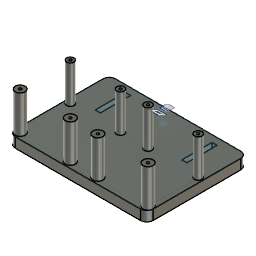
Halterung_BTS7960 (Autodesk Fusion 360 design; units mm, degrees)
part number: 2026-02-15-17-28-29-265
Autodesk Fusion 360 part; units mm, degrees
sketch "Skizze1" plane through (0, 0, 0) normal (0, 0, 1) x (1, 0, 0)
  line L0 (-35, 15) -> (50, 15)
  line L1 (50, 15) -> (50, -20)
  line L2 (50, -20) -> (-35, -20)
  line L3 (-35, -20) -> (-35, 15)
  dimension "d1" = 85
  dimension "d2" = 35
  constraint horizontal L0
  constraint vertical L1
  constraint horizontal L2
  constraint vertical L3
  measures "d1" distance of L0.start L0.end
  measures "d2" distance of L0 L2
extrude "Extrusion1" add sketch "Skizze1" along normal blind 8
sketch "Skizze2" plane through (0, 0, 8) normal (0, 0, 1) x (-1, 0, 0)
  line L0 (35, 20) -> (-50, 20)
  line L1 (-50, 20) -> (-50, -15)
  line L2 (-50, -15) -> (35, -15)
  line L3 (35, -15) -> (35, 20)
  line L4 (29, -9.5) -> (25, -9.5)
  line L5 (25, -9.5) -> (25, 14.5)
  line L6 (25, 14.5) -> (29, 14.5)
  line L7 (29, 14.5) -> (29, -9.5)
  line L8 (-40, -9.5) -> (-44, -9.5)
  line L9 (-44, -9.5) -> (-44, 14.5)
  line L10 (-44, 14.5) -> (-40, 14.5)
  line L11 (-40, 14.5) -> (-40, -9.5)
  dimension "d5" = 65
  dimension "d6" = 6
  dimension "d7" = 6
  dimension "d8" = 4
  dimension "d9" = 4
  dimension "d10" = 5.5
  dimension "d16" = 35
  dimension "d17" = 24
  dimension "d18" = 24
  dimension "d19" = 5.5
  dimension "d20" = 5.5
  constraint horizontal L4
  constraint vertical L5
  constraint horizontal L6
  constraint vertical L7
  constraint horizontal L8
  constraint vertical L9
  constraint horizontal L10
  constraint vertical L11
  measures "d5" distance of L5 L11
  measures "d6" distance of L3 L7
  measures "d7" distance of L1 L9
  measures "d8" distance of L9.end L10.end
  measures "d9" distance of L5.end L6.end
  measures "d10" distance of L0 L6
  measures "d16" distance of L0.start L2.end
  measures "d17" distance of L4 L6
  measures "d18" distance of L8.end L9.end
  measures "d19" distance of L0 L10
  measures "d20" distance of L2 L8
extrude "Extrusion2" cut sketch "Skizze2" against normal blind 8 contours L4 L5 L6 L7 | L8 L9 L10 L11
sketch "Skizze3" plane through (0, 0, 8) normal (0, 0, 1) x (-1, 0, 0)
  line L0 (25, -9.5) -> (25, 14.5)
  line L1 (25, 14.5) -> (29, 14.5)
  line L2 (29, 14.5) -> (29, -9.5)
  line L3 (29, -9.5) -> (25, -9.5)
  line L4 (-44, -9.5) -> (-44, 14.5)
  line L5 (-44, 14.5) -> (-40, 14.5)
  line L6 (-40, 14.5) -> (-40, -9.5)
  line L7 (-40, -9.5) -> (-44, -9.5)
  line L8 (35, 20) -> (-50, 20)
  line L9 (-50, 20) -> (-50, -15)
  line L10 (-50, -15) -> (35, -15)
  line L11 (35, -15) -> (35, 20)
  point P0 (-7.5, -3)
  dimension "d13" = 42.5
  dimension "d14" = 4
  dimension "d15" = 5.5
  dimension "d21" = 12
  measures "d13" distance of L11 P0
  measures "d14" distance of L0.start L2.end
  measures "d15" distance of L3 L10
  measures "d21" distance of L10 P0
hole "Bohrung1" at (7.5, 3, 8) direction (0, 0, -1) diameter 4 depth 25 tip angle 118
sketch "Skizze4" plane through (-35, 0, 0) normal (-1, 0, 0) x (0, -1, 0)
  line L0 (-15, 0) -> (20, 0)
  line L1 (20, 0) -> (20, 8)
  line L2 (20, 8) -> (-15, 8)
  line L3 (-15, 8) -> (-15, 0)
  line L4 (-15, 8) -> (20, 8)
  line L5 (20, 8) -> (20, 0)
  line L6 (20, 0) -> (-15, 0)
  line L7 (-15, 0) -> (-15, 8)
  constraint horizontal L4
  constraint vertical L5
  constraint horizontal L6
  constraint vertical L7
  constraint coincident L0.end L1.start
  constraint coincident L2.end L3.start
extrude "Extrusion3" add sketch "Skizze4" along normal blind 12.5
sketch "Skizze5" plane through (50, 0, 0) normal (1, 0, 0) x (0, 1, 0)
  line L0 (-20, 0) -> (15, 0)
  line L1 (15, 0) -> (15, 8)
  line L2 (15, 8) -> (-20, 8)
  line L3 (-20, 8) -> (-20, 0)
  line L4 (-20, 8) -> (15, 8)
  line L5 (15, 8) -> (15, 0)
  line L6 (15, 0) -> (-20, 0)
  line L7 (-20, 0) -> (-20, 8)
  constraint horizontal L4
  constraint vertical L5
  constraint horizontal L6
  constraint vertical L7
  constraint coincident L0.end L1.start
  constraint coincident L2.end L3.start
extrude "Extrusion4" add sketch "Skizze5" along normal blind 12.5
sketch "Skizze6" plane through (0, 0, 8) normal (0, 0, 1) x (-1, 0, 0)
  circle A0 centre (-7.5, -3) radius 2
  line L0 (25, -9.5) -> (25, 14.5)
  line L1 (25, 14.5) -> (29, 14.5)
  line L2 (29, 14.5) -> (29, -9.5)
  line L3 (29, -9.5) -> (25, -9.5)
  line L4 (-44, -9.5) -> (-44, 14.5)
  line L5 (-44, 14.5) -> (-40, 14.5)
  line L6 (-40, 14.5) -> (-40, -9.5)
  line L7 (-40, -9.5) -> (-44, -9.5)
sketch "Skizze7" plane through (0, -20, 0) normal (0, -1, 0) x (1, 0, 0)
  line L0 (-47.5, 0) -> (62.5, 0)
  line L1 (62.5, 0) -> (62.5, 8)
  line L2 (62.5, 8) -> (-47.5, 8)
  line L3 (-47.5, 8) -> (-47.5, 0)
  line L4 (-47.5, 8) -> (62.5, 8)
  line L5 (62.5, 8) -> (62.5, 0)
  line L6 (62.5, 0) -> (-47.5, 0)
  line L7 (-47.5, 0) -> (-47.5, 8)
  constraint horizontal L4
  constraint vertical L5
  constraint horizontal L6
  constraint vertical L7
  constraint coincident L0.end L1.start
  constraint coincident L2.end L3.start
extrude "Extrusion5" add sketch "Skizze7" along normal blind 45
sketch "Skizze8" plane through (0, 0, 8) normal (0, 0, 1) x (-1, 0, 0)
  line L0 (25, -9.5) -> (25, 14.5)
  line L1 (25, 14.5) -> (29, 14.5)
  line L2 (29, 14.5) -> (29, -9.5)
  line L3 (29, -9.5) -> (25, -9.5)
  line L4 (-44, -9.5) -> (-44, 14.5)
  line L5 (-44, 14.5) -> (-40, 14.5)
  line L6 (-40, 14.5) -> (-40, -9.5)
  line L7 (-40, -9.5) -> (-44, -9.5)
  line L8 (-62.5, 65) -> (-62.5, -15)
  line L9 (-62.5, -15) -> (47.5, -15)
  line L10 (47.5, -15) -> (47.5, 65)
  line L11 (47.5, 65) -> (-62.5, 65)
sketch "Skizze9" plane through (0, 0, 8) normal (0, 0, 1) x (-1, 0, 0)
  line L0 (-62.5, -15) -> (47.5, -15)
  line L1 (47.5, 65) -> (-62.5, 65)
  circle A0 centre (43.5, 60) radius 4
  line L2 (47.5, -15) -> (47.5, 65)
  circle A1 centre (43.5, 20) radius 3
  circle A2 centre (3.5, 20) radius 3
  circle A3 centre (3.5, 60) radius 4
  circle A4 centre (-58.5, 60) radius 4
  circle A5 centre (-58.5, 20) radius 3
  circle A6 centre (-18.5, 20) radius 3
  circle A7 centre (-18.5, 60) radius 4
  line L3 (-62.5, 65) -> (-62.5, -15)
  dimension "d32" = 110
  dimension "d33" = 80
  dimension "d34" = 8
  dimension "d35" = 110
  dimension "d36" = 75
  dimension "d37" = 4
  dimension "d38" = 6
  dimension "d39" = 6
  dimension "d40" = 8
  dimension "d41" = 40
  dimension "d42" = 40
  dimension "d43" = 40
  dimension "d44" = 40
  dimension "d45" = 8
  dimension "d46" = 6
  dimension "d47" = 6
  dimension "d48" = 8
  dimension "d49" = 40
  dimension "d50" = 40
  dimension "d51" = 40
  dimension "d52" = 40
  dimension "d53" = 75
  dimension "d55" = 4
  dimension "d56" = 4
  dimension "d57" = 5
  dimension "d58" = 5
  dimension "d68" = 80
  dimension "d69" = 4
  dimension "d70" = 5
  measures "d32" distance of L0.start L0.end
  measures "d33" distance of L0 L1
  measures "d34" diameter of A0
  measures "d35" distance of L0.start L0.end
  measures "d36" distance of L0 A0.centre
  measures "d37" distance of A0.centre L2
  measures "d38" diameter of A1
  measures "d39" diameter of A2
  measures "d40" diameter of A3
  measures "d41" distance of A0.centre A3.centre
  measures "d42" distance of A0.centre A1.centre
  measures "d43" distance of A2.centre A3.centre
  measures "d44" distance of A1.centre A2.centre
  measures "d45" diameter of A7
  measures "d46" diameter of A6
  measures "d47" diameter of A5
  measures "d48" diameter of A4
  measures "d49" distance of A7.centre A4.centre
  measures "d50" distance of A7.centre A6.centre
  measures "d51" distance of A5.centre A4.centre
  measures "d52" distance of A6.centre A5.centre
  measures "d53" distance of L0 A4.centre
  measures "d55" distance of A4.centre L3
  measures "d56" distance of A5.centre L3
  measures "d57" distance of L1 A4.centre
  measures "d58" distance of L1 A7.centre
  measures "d68" distance of L1.start L0.end
  measures "d69" distance of L2 A1.centre
  measures "d70" distance of L1 A3.centre
extrude "Extrusion6" add sketch "Skizze9" along normal blind 30 contours A0 | A4 | A1 | A2 | A3 | A5 | A6 | A7
sketch "Skizze10" plane through (0, 0, 38) normal (0, 0, 1) x (-1, 0, 0)
  circle A0 centre (43.5, 20) radius 3
  point P0 (43.5, 20)
  point P1 (43.5, 60)
  point P2 (3.5, 30)
  point P3 (3.5, 60)
  point P4 (-18.5, 60)
  point P5 (-18.5, 30)
  point P6 (-58.5, 30)
  point P7 (-58.5, 60)
  constraint coincident P0 A0.centre
hole "Bohrung2" at (-43.5, -20, 38) at (-3.5, -30, 38) at (18.5, -30, 38) at (58.5, -30, 38) at (58.5, -60, 38) at (18.5, -60, 38) at (-3.5, -60, 38) at (-43.5, -60, 38) direction (0, 0, -1) diameter 2 depth 4 tip angle 180
fillet "Abrundung1" radius 5 1 edges at (-47.5, -65, 4)
fillet "Abrundung2" radius 5 3 edges at (62.5, 15, 4) (62.5, -65, 4) (-47.5, 15, 4)
delete_face "Fläche löschen1" 1 faces at (7.6991, 1.0099, 5.3333)
sketch "Skizze11" plane through (0, 0, 38) normal (0, 0, 1) x (-1, 0, 0)
  circle A0 centre (3.5, 20) radius 3
  point P0 (-58.5, 20)
  point P1 (-18.5, 20)
  point P2 (3.5, 20)
  constraint coincident P2 A0.centre
hole "Bohrung3" at (58.5, -20, 38) at (18.5, -20, 38) at (-3.5, -20, 38) direction (0, 0, -1) diameter 2 depth 3 tip angle 180
